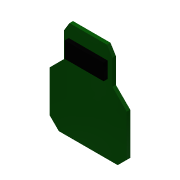
# Autodesk Inventor part: WirebondAdapter
Saved by Autodesk Inventor 2014 (Build 180170000, 170)
## iProperties
Created: 2016-07-07
Part Number: WirebondAdapter
Material: Generic
Document SubType Name: Modeling
Designer: Camilo
Density: 1 g/cm^3
Appearance: LED - Green Off
Author: Camilo
Autodesk Inventor part; units mm, degrees
ref_plane "YZ Plane" through (0, 0, 0) normal (1, 0, 0) x (0, 1, 0)
ref_plane "XZ Plane" through (0, 0, 0) normal (0, 1, 0) x (-1, 0, 0)
ref_plane "XY Plane" through (0, 0, 0) normal (0, 0, 1) x (1, 0, 0)
sketch "Sketch1" plane through (0, 0, 0) normal (0, 1, 0) x (-1, 0, 0)
  line L0 (-6.395, -10.74) -> (6.395, -10.74)
  line L1 (6.395, -10.74) -> (8.355, -8.78)
  line L2 (8.355, -8.78) -> (8.355, 0.28)
  line L3 (8.355, 0.28) -> (5.235, 3.4)
  line L4 (5.235, 3.4) -> (5.235, 8.84)
  line L5 (5.235, 8.84) -> (4.07, 10.74)
  line L6 (-6.395, -10.74) -> (-8.355, -8.78)
  line L7 (-8.355, -8.78) -> (-8.355, 0.28)
  line L8 (-8.355, 0.28) -> (-5.235, 3.4)
  line L9 (-5.235, 3.4) -> (-5.235, 8.84)
  line L10 (-5.235, 8.84) -> (-4.07, 10.74)
  line L11 (-4.07, 10.74) -> (4.07, 10.74)
  dimension "d0" = 12.79
  constraints: 24 end point
  measures "d0" distance of L0.start L0.end
extrude "Extrusion1" add sketch "Sketch1" along normal blind 0.76
sketch "Sketch2" plane through (0, 0.76, 0) normal (0, 1, 0) x (1, 0, 0)
  line L0 (-5.235, -3.4) -> (5.235, -3.4) construction
  line L1 (5.235, -3.4) -> (5.235, -8.84) construction
  line L2 (5.235, -8.84) -> (-5.235, -8.84) construction
  line L3 (-5.235, -8.84) -> (-5.235, -3.4) construction
  line L4 (4.235, -4.4) -> (-4.235, -4.4)
  line L5 (-4.235, -4.4) -> (-4.235, -7.84)
  line L6 (-4.235, -7.84) -> (4.235, -7.84)
  line L7 (4.235, -7.84) -> (4.235, -4.4)
  point P0 (0, 0)
  dimension "d4" = 1
  constraints: 16 end point, 3 other
  measures "d4" distance between parallel lines of L0 L4
extrude "Extrusion2" add sketch "Sketch2" along normal blind 0.9
sketch "Sketch3" plane through (0, 0, 0) normal (0, -1, 0) x (1, 0, 0)
  line L0 (4.235, 4.4) -> (-4.235, 4.4) projected
  line L1 (-4.235, 4.4) -> (-4.235, 7.84) projected
  line L2 (-4.235, 7.84) -> (4.235, 7.84) projected
  line L3 (4.235, 7.84) -> (4.235, 4.4) projected
  point P0 (0, 0)
extrude "Extrusion3" add sketch "Sketch3" along normal blind 0.9
body "Solid1"
